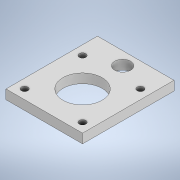
# Autodesk Inventor part: zmotorsupport
Saved by Autodesk Inventor 2020.2 (Build 242310000, 310)
## iProperties
Created: 2020-07-31
Part Number: zmotorsupport
Material: Generic
Document SubType Name: Modeling
Designer: JK
Density: 1 g/cm^3
Appearance: Default
Author: JK
Autodesk Inventor part; units mm, degrees
ref_plane "YZ Plane" through (0, 0, 0) normal (1, 0, 0) x (0, 1, 0)
ref_plane "XZ Plane" through (0, 0, 0) normal (0, 1, 0) x (-1, 0, 0)
ref_plane "XY Plane" through (0, 0, 0) normal (0, 0, 1) x (1, 0, 0)
sketch "Sketch1" plane through (0, 0, 0) normal (0, 1, 0) x (-1, 0, 0)
  circle A0 centre (0, 0) radius 10.5
  circle A1 centre (0, -21.5) radius 4.25
  line L0 (-20.5, 20.5) -> (20.5, 20.5)
  line L1 (20.5, 20.5) -> (20.5, -20.5)
  line L2 (20.5, -20.5) -> (-20.5, -20.5)
  line L3 (-20.5, -20.5) -> (-20.5, 20.5)
  line L4 (-20.5, 20.5) -> (20.5, -20.5) construction
  line L5 (20.5, 20.5) -> (-20.5, -20.5) construction
  line L6 (20.5, -20.5) -> (-20.5, -20.5)
  line L7 (-20.5, -20.5) -> (-20.5, -28.5)
  line L8 (-20.5, -28.5) -> (20.5, -28.5)
  line L9 (20.5, -28.5) -> (20.5, -20.5)
  circle A2 centre (15.5, 15.5) radius 1.75
  circle A3 centre (15.5, -15.5) radius 1.75
  circle A4 centre (-15.5, -15.5) radius 1.75
  circle A5 centre (-15.5, 15.5) radius 1.75
  point P0 (0, 0)
  dimension "d0" = 21
  dimension "d1" = 21.5
  dimension "d2" = 8.5
  dimension "d3" = 41
  dimension "d4" = 41
  dimension "d5" = 3.5
  dimension "d6" = 31
  dimension "d7" = 31
  dimension "d8" = 8
  constraints: 20 end point, 6 centre point, 4 parallel, 4 point on line, 3 equal radius, 3 midpoint, 2 horizontal, 2 horizontal alignment, 2 perpendicular, 2 vertical alignment, 1 coincident
  measures "d0" diameter of A0
  measures "d1" distance of A1.centre point (0, 0)
  measures "d2" diameter of A1
  measures "d3" distance of L0.start L0.end
  measures "d4" distance of L0.end L1.end
  measures "d5" diameter of A3
  measures "d6" distance of A2.centre A3.centre
  measures "d7" distance of A4.centre A3.centre
  measures "d8" distance of L8.end L1.end
extrude "Extrusion1" add sketch "Sketch1" along normal blind 5 contours A1 L2 L9 L8 L7 | A1 L2 L3 L0 L1
body "Solid1"
